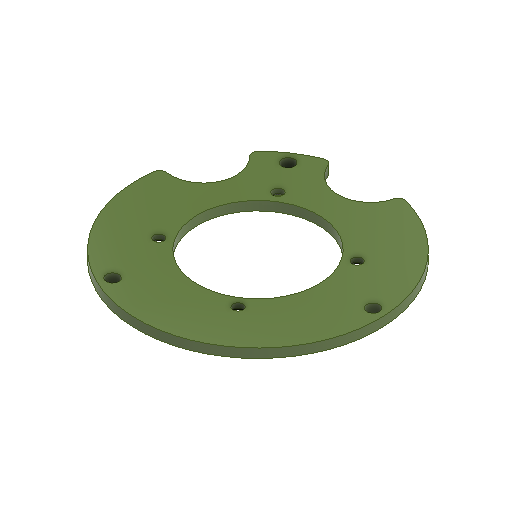
# Autodesk Inventor part: cathode_jig
Saved by Autodesk Inventor 2024.2 (Build 282272000, 272)
## iProperties
Created: 2020-04-09
Part Number: cathode_jig
Material: 一般
Document SubType Name: Modeling
Designer: Yun
Density: 1 g/cm^3
Appearance: Dark Olive
Mass: 9.95986 g
Surface Area: 80.7505 cm^2
Volume: 9.95986 cm^3
Author: Yun
Autodesk Inventor part; units mm, degrees
ref_plane "YZ Plane" through (0, 0, 0) normal (1, 0, 0) x (0, 1, 0)
ref_plane "XZ Plane" through (0, 0, 0) normal (0, 1, 0) x (-1, 0, 0)
ref_plane "XY Plane" through (0, 0, 0) normal (0, 0, 1) x (1, 0, 0)
sketch "スケッチ1" plane through (0, 0, 0) normal (0, 1, 0) x (-1, 0, 0)
  circle A0 centre (0, 0) radius 20
  circle A1 centre (0, 0) radius 40
  dimension "d0" = 40
  dimension "OD" = 80
  constraints: 2 centre point, 2 coincident
  measures "d0" diameter of A0
  measures "OD" diameter of A1
extrude "押し出し1" add sketch "スケッチ1" along normal blind 3
sketch "スケッチ8" plane through (0, 0, 0) normal (0, -1, 0) x (1, 0, 0)
  circle A0 centre (-0.0001, 0) radius 23.75
  circle A1 centre (-27.2635, 37.05) radius 3.15 projected
  circle A2 centre (-38.2912, 25.4909) radius 3.15 projected
  circle A3 centre (25.4909, 38.2912) radius 5.525 projected
  circle A4 centre (41.2214, 20.4157) radius 5.525 projected
  circle A5 centre (38.2912, -25.4909) radius 4.65 projected
  circle A6 centre (-35.8447, -17.7527) radius 4.65 projected
  circle A7 centre (-2.548, -39.9188) radius 4.65 projected
  arc A8 (-4.7957, -75.1327) -> (4.7957, 75.1327) centre (0, 0) ccw projected
  arc A9 (4.7957, 75.1327) -> (-4.7957, -75.1327) centre (0, 0) ccw projected
  circle A10 centre (-16.7482, -62.9346) radius 4.2164 projected
  circle A11 centre (-39.5574, -51.7347) radius 4.2164 projected
  circle A12 centre (-56.3443, -32.6587) radius 4.2164 projected
  circle A13 centre (-64.5532, -8.6107) radius 4.2164 projected
  circle A14 centre (-62.9346, 16.7482) radius 4.2164 projected
  circle A15 centre (-51.7347, 39.5574) radius 4.2164 projected
  circle A16 centre (-32.6587, 56.3443) radius 4.2164 projected
  circle A17 centre (-8.6107, 64.5532) radius 4.2164 projected
  circle A18 centre (16.7482, 62.9346) radius 4.2164 projected
  circle A19 centre (39.5574, 51.7347) radius 4.2164 projected
  circle A20 centre (56.3443, 32.6587) radius 4.2164 projected
  circle A21 centre (64.5532, 8.6107) radius 4.2164 projected
  circle A22 centre (62.9346, -16.7482) radius 4.2164 projected
  circle A23 centre (51.7347, -39.5574) radius 4.2164 projected
  circle A24 centre (32.6587, -56.3443) radius 4.2164 projected
  circle A25 centre (8.6107, -64.5532) radius 4.2164 projected
  circle A26 centre (-29.3091, 1.8708) radius 2.7051 projected
  circle A27 centre (-16.2747, -24.447) radius 2.7051 projected
  circle A28 centre (13.0344, -26.3178) radius 2.7051 projected
  circle A29 centre (29.3091, -1.8708) radius 2.7051 projected
  circle A30 centre (16.2747, 24.447) radius 2.7051 projected
  circle A31 centre (-13.0344, 26.3178) radius 2.7051 projected
  ellipse E0 centre (0.0001, 0) end of major axis (24.6134, -1.5711) minor radius 24.6634 (1.5711, 24.6133) -> (-1.5711, -24.6133) ccw projected
  ellipse E1 centre (-0.0001, 0) end of major axis (24.6133, -1.5711) minor radius 24.6634 (-1.5711, -24.6133) -> (1.5711, 24.6133) ccw projected
  line L0 (-16.2747, -24.447) -> (-0.0001, 0) construction
  line L1 (19.7699, -13.161) -> (-19.77, 13.161) construction
  point P0 (13.161, 19.7699)
  point P1 (-13.1611, -19.7699)
  dimension "d88" = 47.5
  constraints: 4 end point, 4 point on circle, 2 coincident, 2 point on line, 1 centre point, 1 midpoint, 1 perpendicular, 2 other
  measures "d88" diameter of A0
hole "穴3" at (-19.77, 0, 13.161) at (13.161, 0, 19.7699) at (19.7699, 0, -13.161) at (-13.1611, 0, -19.7699) direction (0, 1, 0) diameter 3.4 depth 3 countersink diameter 6.3 countersink angle 90
sketch "Sketch11" plane through (0, 3, 0) normal (0, 1, 0) x (1, 0, 0)
  circle A0 centre (-2.548, 39.9188) radius 6.6 projected
  circle A1 centre (-35.8447, 17.7527) radius 6.858 projected
  circle A2 centre (-35.8447, 17.7527) radius 10.858
  circle A3 centre (-2.548, 39.9188) radius 10.858
  point P0 (0, 0)
  dimension "d71" = 4
  constraints: 2 centre point, 2 coincident, 1 equal radius
  measures "d71" radial gap between concentric circles of A1 A2
extrude "Extrusion5" cut sketch "Sketch11" against normal through all contours A0 | A1 | A2 | A3
sketch "Sketch13" plane through (0, 3, 0) normal (0, 1, 0) x (1, 0, 0)
  circle A0 centre (-19.9494, 29.967) radius 2.1
  circle A1 centre (35.9269, 2.2932) radius 2.1
  circle A2 centre (-15.9775, -32.2602) radius 2.1
  circle A3 centre (0, 0) radius 36 construction
  arc A4 (-13.1898, 37.7628) -> (8.2815, 39.1333) centre (-2.548, 39.9188) ccw projected
  arc A5 (-39.2984, 7.4587) -> (-29.7497, 26.7387) centre (-35.8447, 17.7527) ccw projected
  line L0 (-2.548, 39.9188) -> (-35.8447, 17.7527) construction
  line L1 (-19.1963, 28.8358) -> (0, 0) construction
  line L2 (0, 0) -> (35.9269, 2.2932) construction
  line L3 (0, 0) -> (-15.9775, -32.2602) construction
  dimension "d83" = 72
  dimension "d84" = 4.2
  dimension "d85" = 120
  dimension "d86" = 120
  constraints: 8 end point, 4 centre point, 3 point on circle, 2 equal radius, 1 coincident, 1 midpoint, 1 point on line
  measures "d83" diameter of A3
  measures "d84" diameter of A0
  measures "d85" angle of L2 L1
  measures "d86" angle of L3 L1
extrude "Extrusion7" cut sketch "Sketch13" against normal through all
fillet "Fillet2" radius 2 4 edges at (-39.2984, 1.5, -7.4587) (-29.7497, 1.5, -26.7387) (8.2815, 1.5, -39.1333) (-13.1898, 1.5, -37.7628)
